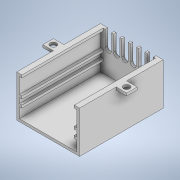
# Autodesk Inventor part: main
Saved by Autodesk Inventor 2021 (Build 250183000, 183)
## iProperties
Created: 2021-01-26
Part Number: main
Material: Generic
Document SubType Name: Modeling
Designer: Ryan
Density: 1 g/cm^3
Appearance: Default
Author: Ryan
Autodesk Inventor part; units mm, degrees
ref_plane "YZ Plane" through (0, 0, 0) normal (1, 0, 0) x (0, 1, 0)
ref_plane "XZ Plane" through (0, 0, 0) normal (0, 1, 0) x (-1, 0, 0)
ref_plane "XY Plane" through (0, 0, 0) normal (0, 0, 1) x (1, 0, 0)
sketch "Sketch1" plane through (0, 0, 0) normal (0, 1, 0) x (-1, 0, 0)
  line L0 (38.1, 50.8) -> (-38.1, 50.8)
  line L1 (-38.1, 50.8) -> (-38.1, -50.8)
  line L2 (-38.1, -50.8) -> (38.1, -50.8)
  line L3 (38.1, -50.8) -> (38.1, 50.8)
  point P0 (0, 0)
  dimension "d0" = 101.6
  dimension "d1" = 76.2
  dimension "d2" = 38.1
  dimension "d3" = 50.8
  constraints: 8 end point, 2 parallel, 1 horizontal, 1 perpendicular
  measures "d0" distance of L2.end L0.start
  measures "d1" distance of L0.start L0.end
  measures "d2" distance from line of point (0, 0) L3
  measures "d3" distance from line of point (0, 0) L0
extrude "Extrusion1" add sketch "Sketch1" along normal blind 50.8
sketch "Sketch2" plane through (-38.1, 0, 50.8) normal (0, 0, 1) x (1, 0, 0)
  line L0 (76.2, 50.8) -> (0, 50.8) projected
  line L1 (76.2, 0) -> (0, 0) projected
  line L2 (0, 50.8) -> (3.175, 50.8)
  line L3 (3.175, 50.8) -> (3.175, 0)
  line L4 (0, 0) -> (0, 50.8)
  line L5 (76.2, 0) -> (76.2, 50.8) projected
  line L6 (0, 50.8) -> (76.2, 50.8)
  line L7 (76.2, 50.8) -> (76.2, 47.625)
  line L8 (0, 47.625) -> (0, 50.8)
  line L9 (76.2, 50.8) -> (73.025, 50.8)
  line L10 (73.025, 50.8) -> (73.025, 0)
  line L11 (76.2, 0) -> (76.2, 50.8)
  line L12 (3.175, 15.875) -> (6.35, 15.875)
  line L13 (6.35, 15.875) -> (6.35, 19.05)
  line L14 (6.35, 19.05) -> (3.175, 19.05)
  line L15 (3.175, 19.05) -> (3.175, 15.875)
  line L16 (3.175, 25.4) -> (6.35, 25.4)
  line L17 (6.35, 25.4) -> (6.35, 28.575)
  line L18 (6.35, 28.575) -> (3.175, 28.575)
  line L19 (3.175, 28.575) -> (3.175, 25.4)
  line L20 (38.1, 47.625) -> (38.1, 0)
  line L21 (73.025, 15.875) -> (69.85, 15.875)
  line L22 (69.85, 15.875) -> (69.85, 19.05)
  line L23 (69.85, 19.05) -> (73.025, 19.05)
  line L24 (73.025, 25.4) -> (69.85, 25.4)
  line L25 (69.85, 25.4) -> (69.85, 28.575)
  line L26 (69.85, 28.575) -> (73.025, 28.575)
  line L27 (3.175, 50.8) -> (6.35, 50.8)
  line L28 (6.35, 50.8) -> (6.35, 47.625)
  line L29 (6.35, 47.625) -> (3.175, 47.625)
  line L30 (3.175, 47.625) -> (3.175, 50.8)
  line L31 (73.025, 50.8) -> (69.85, 50.8)
  line L32 (69.85, 50.8) -> (69.85, 47.625)
  line L33 (69.85, 47.625) -> (73.025, 47.625)
  line L34 (73.025, 47.625) -> (73.025, 50.8)
  line L35 (0, 0) -> (76.2, 0)
  line L36 (76.2, 0) -> (76.2, 3.175)
  line L37 (76.2, 3.175) -> (0, 3.175)
  line L38 (0, 3.175) -> (0, 0)
  point P0 (3.175, 3.175)
  point P1 (73.025, 3.175)
  point P2 (6.35, 50.8)
  point P3 (3.175, 47.625)
  point P4 (3.175, 28.575)
  point P5 (3.175, 19.05)
  dimension "d6" = 3.175
  dimension "d8" = 3.175
  dimension "d11" = 3.175
  dimension "d12" = 3.175
  dimension "d13" = 3.175
  dimension "d15" = 6.35
  dimension "d16" = 3.175
  dimension "d17" = 12.7
  dimension "d18" = 0
  constraints: 72 end point, 13 parallel, 8 horizontal, 8 perpendicular, 8 symmetric about line, 7 point on line, 1 midpoint, 1 vertical
  measures "d6" distance between parallel lines of L4 L3
  measures "d8" distance between parallel lines of L5 L10
  measures "d11" distance of L17.end L18.end
  measures "d12" distance of L12.end L13.end
  measures "d13" distance of L16.end L17.end
  measures "d15" distance between parallel lines of L16 L14
  measures "d16" distance between parallel lines of L35 L37
  measures "d17" distance between parallel lines of L37 L12
  measures "d18" distance between parallel lines of L1 L35
extrude "Extrusion2" cut sketch "Sketch2" against normal blind 98.425 contours L32 L33 L10 L26 L25 L24 L23 L22 L21 L37 L3 L12 L13 L14 L16 L17 L18 L29 L28 L0
sketch "Sketch3" plane through (38.1, 0, -50.8) normal (0, 0, -1) x (-1, 0, 0)
  line L0 (0, 50.8) -> (76.2, 50.8) projected
  line L1 (38.1, 0) -> (38.1, 50.8) construction
  line L2 (29.21, 50.8) -> (36.83, 50.8)
  line L3 (36.83, 50.8) -> (36.83, 31.75)
  line L4 (29.21, 31.75) -> (29.21, 50.8)
  line L5 (26.67, 50.8) -> (19.05, 50.8)
  line L6 (19.05, 50.8) -> (19.05, 31.75)
  line L7 (26.67, 31.75) -> (26.67, 50.8)
  line L8 (33.02, 31.75) -> (33.02, 50.8) construction
  line L9 (22.86, 31.75) -> (22.86, 50.8) construction
  line L10 (16.51, 50.8) -> (8.89, 50.8)
  line L11 (8.89, 50.8) -> (8.89, 31.75)
  line L12 (16.51, 31.75) -> (16.51, 50.8)
  line L13 (12.7, 31.75) -> (12.7, 50.8) construction
  arc A0 (8.89, 31.75) -> (16.51, 31.75) centre (12.7, 31.75) ccw
  arc A1 (19.05, 31.75) -> (26.67, 31.75) centre (22.86, 31.75) ccw
  arc A2 (29.21, 31.75) -> (36.83, 31.75) centre (33.02, 31.75) ccw
  line L14 (8.89, 31.75) -> (36.83, 31.75) construction
  line L15 (46.99, 50.8) -> (39.37, 50.8)
  line L16 (39.37, 50.8) -> (39.37, 31.75)
  line L17 (46.99, 31.75) -> (46.99, 50.8)
  line L18 (49.53, 50.8) -> (57.15, 50.8)
  line L19 (57.15, 50.8) -> (57.15, 31.75)
  line L20 (49.53, 31.75) -> (49.53, 50.8)
  line L21 (43.18, 31.75) -> (43.18, 50.8) construction
  line L22 (53.34, 31.75) -> (53.34, 50.8) construction
  line L23 (59.69, 50.8) -> (67.31, 50.8)
  line L24 (67.31, 50.8) -> (67.31, 31.75)
  line L25 (59.69, 31.75) -> (59.69, 50.8)
  line L26 (63.5, 31.75) -> (63.5, 50.8) construction
  arc A3 (59.69, 31.75) -> (67.31, 31.75) centre (63.5, 31.75) ccw
  arc A4 (49.53, 31.75) -> (57.15, 31.75) centre (53.34, 31.75) ccw
  arc A5 (39.37, 31.75) -> (46.99, 31.75) centre (43.18, 31.75) ccw
  line L27 (67.31, 31.75) -> (39.37, 31.75) construction
  point P0 (19.05, 50.8)
  point P1 (8.89, 50.8)
  dimension "d21" = 10.16
  dimension "d22" = 5.08
  dimension "d24" = 7.62
  dimension "d25" = 7.62
  dimension "d26" = 10.16
  dimension "d27" = 7.62
  dimension "d28" = 19.05
  constraints: 54 end point, 21 symmetric about line, 12 point on circle, 7 point on line, 6 centre point, 6 coincident, 6 midpoint, 6 parallel, 4 perpendicular, 3 horizontal, 3 other
  measures "d21" distance between parallel lines of L9 L8
  measures "d22" distance between parallel lines of L1 L8
  measures "d24" distance between parallel lines of L4 L3
  measures "d25" distance between parallel lines of L6 L7
  measures "d26" distance between parallel lines of L9 L13
  measures "d27" distance between parallel lines of L11 L12
  measures "d28" distance of L10.end L11.end
extrude "Extrusion3" cut sketch "Sketch3" against normal blind 3.175
sketch "Sketch4" plane through (38.1, 0, 50.8) normal (1, 0, 0) x (0, 0, -1)
  line L0 (50.8, 0) -> (50.8, 50.8) construction
  line L1 (0, 50.8) -> (101.6, 50.8) projected
  line L2 (44.45, 50.8) -> (57.15, 50.8)
  line L3 (57.15, 50.8) -> (57.15, 47.625)
  line L4 (57.15, 47.625) -> (44.45, 47.625)
  line L5 (44.45, 47.625) -> (44.45, 50.8)
  point P0 (57.15, 50.8)
  dimension "d31" = 3.175
  dimension "d32" = 12.7
  dimension "d33" = 6.35
  constraints: 10 end point, 2 parallel, 1 horizontal, 1 midpoint, 1 perpendicular, 1 point on line
  measures "d31" distance of L4.end L2.start
  measures "d32" distance of L3.end L4.end
  measures "d33" distance between parallel lines of L0 L5
extrude "Extrusion4" add sketch "Sketch4" along normal blind 12.7
sketch "Sketch5" plane through (-38.1, 0, -50.8) normal (-1, 0, 0) x (0, 0, 1)
  line L0 (50.8, 0) -> (50.8, 50.8) construction
  line L1 (44.45, 50.8) -> (57.15, 50.8)
  line L2 (57.15, 50.8) -> (57.15, 47.625)
  line L3 (57.15, 47.625) -> (44.45, 47.625)
  line L4 (44.45, 47.625) -> (44.45, 50.8)
  dimension "d36" = 3.175
  dimension "d37" = 12.7
  dimension "d38" = 6.35
  constraints: 10 end point, 2 parallel, 1 horizontal, 1 perpendicular
  measures "d36" distance of L3.end L1.start
  measures "d37" distance of L2.end L3.end
  measures "d38" distance between parallel lines of L0 L4
extrude "Extrusion5" add sketch "Sketch5" along normal blind 12.7
sketch "Sketch6" plane through (-38.1, 47.625, -6.35) normal (0, -1, 0) x (1, 0, 0)
  line L0 (0, 0) -> (-12.7, 0) projected
  line L1 (-6.35, 0) -> (-6.35, 12.7) construction
  line L2 (0, 12.7) -> (-12.7, 12.7) projected
  circle A0 centre (-6.35, 6.35) radius 3.81
  point P0 (38.1, 6.35)
  dimension "d41" = 7.62
  constraints: 3 midpoint, 2 end point, 1 centre point
  measures "d41" diameter of A0
extrude "Extrusion6" cut sketch "Sketch6" against normal blind 12.7
sketch "Sketch7" plane through (38.1, 47.625, -6.35) normal (0, -1, 0) x (1, 0, 0)
  line L0 (0, 12.7) -> (12.7, 12.7) projected
  line L1 (6.35, 12.7) -> (6.35, 0) construction
  line L2 (0, 0) -> (12.7, 0) projected
  circle A0 centre (6.35, 6.35) radius 3.81
  point P0 (-38.1, 6.35)
  dimension "d44" = 7.62
  constraints: 3 midpoint, 2 end point, 1 centre point
  measures "d44" diameter of A0
extrude "Extrusion7" cut sketch "Sketch7" against normal blind 12.7
equation "\"d2\" = 0.5 * d1"
equation "\"d3\" = 0.5 * d0"
equation "\"d8\" = d6"
equation "\"d11\" = d6"
equation "\"d12\" = d6"
equation "\"d13\" = d6"
equation "\"d33\" = 0.5 * d32"
equation "\"d38\" = 0.5 * d37"
body "Solid1"
